Autodesk Fusion 360 part; units mm, degrees
(part 2 of 2)
  point P4 (-72.3362, -41.0103)
  point P5 (-72.5298, -38.3408)
  point P6 (-69.8362, -41.0103)
  point P7 (-69.7968, -38.5103)
  point P8 (-69.7968, -41.0103)
  point P9 (-69.9904, -38.3408)
  point P10 (-67.2968, -41.0103)
  point P11 (-67.2573, -38.5103)
  point P12 (-67.2573, -41.0103)
  point P13 (-67.4509, -38.3408)
  point P14 (-64.7573, -41.0103)
  point P15 (-64.7178, -38.5103)
  point P16 (-64.7178, -41.0103)
  point P17 (-64.9114, -38.3408)
  point P18 (-62.2178, -41.0103)
  point P19 (-62.1783, -38.5103)
  point P20 (-62.1783, -41.0103)
  point P21 (-62.3719, -38.3408)
  point P22 (-59.6783, -41.0103)
  point P23 (-59.6389, -38.5103)
  point P24 (-59.6389, -41.0103)
  point P25 (-59.8325, -38.3408)
  point P26 (-57.1389, -41.0103)
  point P27 (-57.0994, -38.5103)
  point P28 (-57.0994, -41.0103)
  point P29 (-57.293, -38.3408)
  point P30 (-54.5994, -41.0103)
  point P31 (-54.5599, -38.5103)
  point P32 (-54.5599, -41.0103)
  point P33 (-54.7535, -38.3408)
  point P34 (-52.0599, -41.0103)
  point P35 (-52.0204, -38.5103)
  point P36 (-52.0204, -41.0103)
  point P37 (-52.214, -38.3408)
  point P38 (-49.5204, -41.0103)
  point P39 (-49.481, -38.5103)
  point P40 (-49.481, -41.0103)
  point P41 (-49.6746, -38.3408)
  point P42 (-46.981, -41.0103)
  point P43 (-46.9415, -38.5103)
  point P44 (-46.9415, -41.0103)
  point P45 (-47.1351, -38.3408)
  point P46 (-44.4415, -41.0103)
  point P47 (-44.402, -38.5103)
  point P48 (-44.402, -41.0103)
  point P49 (-44.5956, -38.3408)
  point P50 (-41.902, -41.0103)
  point P51 (-41.8626, -38.5103)
  point P52 (-41.8626, -41.0103)
  point P53 (-42.0562, -38.3408)
  point P54 (-39.3626, -41.0103)
  point P55 (-39.3231, -38.5103)
  point P56 (-39.3231, -41.0103)
  point P57 (-39.5167, -38.3408)
  point P58 (-36.8231, -41.0103)
  point P59 (-36.7836, -38.5103)
  point P60 (-36.7836, -41.0103)
  point P61 (-36.9772, -38.3408)
  point P62 (-34.2836, -41.0103)
  point P63 (-34.2441, -38.5103)
  point P64 (-34.2441, -41.0103)
  point P65 (-34.4377, -38.3408)
  point P66 (-31.7441, -41.0103)
  point P67 (-31.7047, -38.5103)
  point P68 (-31.7047, -41.0103)
  point P69 (-31.8983, -38.3408)
  point P70 (-29.2047, -41.0103)
  point P71 (-29.1652, -38.5103)
  point P72 (-29.1652, -41.0103)
  point P73 (-29.3588, -38.3408)
  point P74 (-26.6652, -41.0103)
  point P75 (-26.6257, -38.5103)
  point P76 (-26.6257, -41.0103)
  point P77 (-26.8193, -38.3408)
  point P78 (-24.1257, -41.0103)
  point P79 (-74.8757, -53.8103)
  point P80 (-74.8757, -56.3103)
  point P81 (-75.0693, -53.6408)
  point P82 (-72.3757, -56.3103)
  point P83 (-72.3362, -53.8103)
  point P84 (-72.3362, -56.3103)
  point P85 (-72.5298, -53.6408)
  point P86 (-69.8362, -56.3103)
  point P87 (-69.7968, -53.8103)
  point P88 (-69.7968, -56.3103)
  point P89 (-69.9904, -53.6408)
  point P90 (-67.2968, -56.3103)
  point P91 (-67.2573, -53.8103)
  point P92 (-67.2573, -56.3103)
  point P93 (-67.4509, -53.6408)
  point P94 (-64.7573, -56.3103)
  point P95 (-64.7178, -53.8103)
  point P96 (-64.7178, -56.3103)
  point P97 (-64.9114, -53.6408)
  point P98 (-62.2178, -56.3103)
  point P99 (-62.1783, -53.8103)
  point P100 (-62.1783, -56.3103)
  point P101 (-62.3719, -53.6408)
  point P102 (-59.6783, -56.3103)
  point P103 (-59.6389, -53.8103)
  point P104 (-59.6389, -56.3103)
  point P105 (-59.8325, -53.6408)
  point P106 (-57.1389, -56.3103)
  point P107 (-57.0994, -53.8103)
  point P108 (-57.0994, -56.3103)
  point P109 (-57.293, -53.6408)
  point P110 (-54.5994, -56.3103)
  point P111 (-54.5599, -53.8103)
  point P112 (-54.5599, -56.3103)
  point P113 (-54.7535, -53.6408)
  point P114 (-52.0599, -56.3103)
  point P115 (-52.0204, -53.8103)
  point P116 (-52.0204, -56.3103)
  point P117 (-52.214, -53.6408)
  point P118 (-49.5204, -56.3103)
  point P119 (-49.481, -53.8103)
  point P120 (-49.481, -56.3103)
  point P121 (-49.6746, -53.6408)
  point P122 (-46.981, -56.3103)
  point P123 (-46.9415, -53.8103)
  point P124 (-46.9415, -56.3103)
  point P125 (-47.1351, -53.6408)
  point P126 (-44.4415, -56.3103)
  point P127 (-44.402, -53.8103)
  point P128 (-44.402, -56.3103)
  point P129 (-44.5956, -53.6408)
  point P130 (-41.902, -56.3103)
  point P131 (-41.8626, -53.8103)
  point P132 (-41.8626, -56.3103)
  point P133 (-42.0562, -53.6408)
  point P134 (-39.3626, -56.3103)
  point P135 (-39.3231, -53.8103)
  point P136 (-39.3231, -56.3103)
  point P137 (-39.5167, -53.6408)
  point P138 (-36.8231, -56.3103)
  point P139 (-36.7836, -53.8103)
  point P140 (-36.7836, -56.3103)
  point P141 (-36.9772, -53.6408)
  point P142 (-34.2836, -56.3103)
  point P143 (-34.2441, -53.8103)
  point P144 (-34.2441, -56.3103)
  point P145 (-34.4377, -53.6408)
  point P146 (-31.7441, -56.3103)
  point P147 (-31.7047, -53.8103)
  point P148 (-31.7047, -56.3103)
  point P149 (-31.8983, -53.6408)
  point P150 (-29.2047, -56.3103)
  point P151 (-29.1652, -53.8103)
  point P152 (-29.1652, -56.3103)
  point P153 (-29.3588, -53.6408)
  point P154 (-26.6652, -56.3103)
  point P155 (-26.6257, -53.8103)
  point P156 (-26.6257, -56.3103)
  point P157 (-26.8193, -53.6408)
  point P158 (-24.1257, -56.3103)
  dimension "d61" = 2.5
  dimension "d62" = 2.5
  dimension "d63" = -0.7734
  dimension "d64" = 0.5
  dimension "d67" = 48.25
  dimension "d68" = -15.3
  constraint horizontal L4
  constraint vertical L5
  constraint horizontal L6
  constraint vertical L7
  constraint coincident P2 L6
  constraint coincident P2 L7
  constraint tangent L6 A0
  constraint tangent L7 A0
  constraint tangent L5 A1
  constraint tangent L6 A1
  constraint equal A0 A1
  constraint coincident P1 L4
  constraint coincident P1 L5
  constraint tangent L4 A2
  constraint tangent L5 A2
  constraint equal A0 A2
  constraint coincident P0 L4
  constraint coincident P0 L7
  constraint tangent L4 A3
  constraint tangent L7 A3
  constraint equal A0 A3
  measures "d61" distance of P0 P1
  measures "d62" distance of P0 P2
  measures "d64" radius of A0
extrude "Extrude9" add sketch "Sketch5" along normal blind 2.23 separate body contours L4 L5 L6 L7 A0 A1 A2 A3 | A4 L12 L13 A5 A6 L16 A7 L19 | A8 L20 L21 A9 A10 L24 A11 L27 | A12 L28 L29 A13 A14 L32 A15 L35 | A16 L36 L37 A17 A18 L40 A19 L43 | A20 L44 L45 A21 A22 L48 A23 L51 | A24 L52 L53 A25 A26 L56 A27 L59 | A28 L60 L61 A29 A30 L64 A31 L67 | A32 L68 L69 A33 A34 L72 A35 L75 | A36 L76 L77 A37 A38 L80 A39 L83 | A40 L84 L85 A41 A42 L88 A43 L91 | A44 L92 L93 A45 A46 L96 A47 L99 | A48 L100 L101 A49 A50 L104 A51 L107 | A52 L108 L109 A53 A54 L112 A55 L115 | A56 L116 L117 A57 A58 L120 A59 L123 | A60 L124 L125 A61 A62 L128 A63 L131 | A64 L132 L133 A65 A66 L136 A67 L139 | A68 L140 L141 A69 A70 L144 A71 L147 | A72 L148 L149 A73 A74 L152 A75 L155 | A76 L156 L157 A77 A78 L160 A79 L163 | A80 L164 L165 A81 A82 L168 A83 L171 | A84 L172 L173 A85 A86 L176 A87 L179 | A88 L180 L181 A89 A90 L184 A91 L187 | A92 L188 L189 A93 A94 L192 A95 L195 | A96 L196 L197 A97 A98 L200 A99 L203 | A100 L204 L205 A101 A102 L208 A103 L211 | A104 L212 L213 A105 A106 L216 A107 L219 | A108 L220 L221 A109 A110 L224 A111 L227 | A112 L228 L229 A113 A114 L232 A115 L235 | A116 L236 L237 A117 A118 L240 A119 L243 | A120 L244 L245 A121 A122 L248 A123 L251 | A124 L252 L253 A125 A126 L256 A127 L259 | A128 L260 L261 A129 A130 L264 A131 L267 | A132 L268 L269 A133 A134 L272 A135 L275 | A136 L276 L277 A137 A138 L280 A139 L283 | A140 L284 L285 A141 A142 L288 A143 L291 | A144 L292 L293 A145 A146 L296 A147 L299 | A148 L300 L301 A149 A150 L304 A151 L307 | A152 L308 L309 A153 A154 L312 A155 L315 | A156 L316 L317 A157 A158 L320 A159 L323 makes body 21 at (-69.539, 39.6015, 0) makes body 22 at (-59.3811, 39.6015, 0) makes body 23 at (-48.0721, 38.7682, 0) makes body 24 at (-39.0653, 39.6015, 0) makes body 25 at (-28.074, 38.7682, 0) makes body 26 at (-31.4469, 54.9015, 0) makes body 27 at (-41.6047, 54.9015, 0) makes body 28 at (-49.7783, 54.9015, 0) makes body 29 at (-61.9205, 54.9015, 0) makes body 30 at (-72.0784, 54.9015, 0) makes body 31 at (-69.539, 54.9015, 0) makes body 32 at (-59.3811, 54.9015, 0) makes body 33 at (-47.2388, 54.9015, 0) makes body 34 at (-39.0653, 54.9015, 0) makes body 35 at (-28.9074, 54.9015, 0) makes body 36 at (-30.6135, 38.7682, 0) makes body 37 at (-40.7714, 38.7682, 0) makes body 38 at (-49.7783, 39.6015, 0) makes body 39 at (-61.9205, 39.6015, 0) makes body 40 at (-72.0784, 39.6015, 0) makes body 41 at (-66.9995, 39.6015, 0) makes body 42 at (-56.0083, 38.7682, 0) makes body 43 at (-44.6993, 39.6015, 0) makes body 44 at (-36.5258, 39.6015, 0) makes body 45 at (-25.5346, 38.7682, 0) makes body 46 at (-33.9863, 54.9015, 0) makes body 47 at (-44.1442, 54.9015, 0) makes body 48 at (-54.3021, 54.9015, 0) makes body 49 at (-64.46, 54.9015, 0) makes body 50 at (-74.6179, 54.9015, 0) makes body 51 at (-66.9995, 54.9015, 0) makes body 52 at (-56.8416, 54.9015, 0) makes body 53 at (-44.6993, 54.9015, 0) makes body 54 at (-36.5258, 54.9015, 0) makes body 55 at (-26.3679, 54.9015, 0) makes body 56 at (-33.9863, 39.6015, 0) makes body 57 at (-44.1442, 39.6015, 0) makes body 58 at (-54.3021, 39.6015, 0) makes body 59 at (-64.46, 39.6015, 0) makes body 60 at (-74.6179, 39.6015, 0)
extrude "Extrude10" add sketch "Sketch5" along normal blind 8.5 separate body contours L8 L9 L10 L11 | L14 L15 L17 L18 | L22 L23 L25 L26 | L30 L31 L33 L34 | L38 L39 L41 L42 | L46 L47 L49 L50 | L54 L55 L57 L58 | L62 L63 L65 L66 | L70 L71 L73 L74 | L78 L79 L81 L82 | L86 L87 L89 L90 | L94 L95 L97 L98 | L102 L103 L105 L106 | L110 L111 L113 L114 | L118 L119 L121 L122 | L126 L127 L129 L130 | L134 L135 L137 L138 | L142 L143 L145 L146 | L150 L151 L153 L154 | L158 L159 L161 L162 | L166 L167 L169 L170 | L174 L175 L177 L178 | L182 L183 L185 L186 | L190 L191 L193 L194 | L198 L199 L201 L202 | L206 L207 L209 L210 | L214 L215 L217 L218 | L222 L223 L225 L226 | L230 L231 L233 L234 | L238 L239 L241 L242 | L246 L247 L249 L250 | L254 L255 L257 L258 | L262 L263 L265 L266 | L270 L271 L273 L274 | L278 L279 L281 L282 | L286 L287 L289 L290 | L294 L295 L297 L298 | L302 L303 L305 L306 | L310 L311 L313 L314 | L318 L319 L321 L322 makes body 61 at (-29.9781, 39.9192, -2.8333) makes body 62 at (-40.136, 39.9192, -2.8333) makes body 63 at (-50.2939, 39.9192, -2.8333) makes body 64 at (-60.4518, 39.9192, -2.8333) makes body 65 at (-70.6097, 39.9192, -2.8333) makes body 66 at (-68.0702, 55.2192, -2.8333) makes body 67 at (-57.9123, 55.2192, -2.8333) makes body 68 at (-47.7544, 55.2192, -2.8333) makes body 69 at (-37.5965, 55.2192, -2.8333) makes body 70 at (-27.4386, 55.2192, -2.8333) makes body 71 at (-29.9781, 55.2192, -2.8333) makes body 72 at (-40.136, 55.2192, -2.8333) makes body 73 at (-50.2939, 55.2192, -2.8333) makes body 74 at (-60.4518, 55.2192, -2.8333) makes body 75 at (-70.6097, 55.2192, -2.8333) makes body 76 at (-68.0702, 39.9192, -2.8333) makes body 77 at (-57.9123, 39.9192, -2.8333) makes body 78 at (-47.7544, 39.9192, -2.8333) makes body 79 at (-37.5965, 39.9192, -2.8333) makes body 80 at (-27.4386, 39.9192, -2.8333) makes body 81 at (-32.5176, 39.9192, -2.8333) makes body 82 at (-42.6755, 39.9192, -2.8333) makes body 83 at (-52.8333, 39.9192, -2.8333) makes body 84 at (-62.9912, 39.9192, -2.8333) makes body 85 at (-74.1023, 39.6015, -2.8333) makes body 86 at (-65.5307, 55.2192, -2.8333) makes body 87 at (-55.3728, 55.2192, -2.8333) makes body 88 at (-45.2149, 55.2192, -2.8333) makes body 89 at (-35.057, 55.2192, -2.8333) makes body 90 at (-24.8991, 55.2192, -2.8333) makes body 91 at (-32.5176, 55.2192, -2.8333) makes body 92 at (-42.6755, 55.2192, -2.8333) makes body 93 at (-52.8333, 55.2192, -2.8333) makes body 94 at (-62.9912, 55.2192, -2.8333) makes body 95 at (-73.1491, 55.2192, -2.8333) makes body 96 at (-65.5307, 39.9192, -2.8333) makes body 97 at (-55.3728, 39.9192, -2.8333) makes body 98 at (-45.2149, 39.9192, -2.8333) makes body 99 at (-35.057, 39.9192, -2.8333) makes body 100 at (-24.8991, 39.9192, -2.8333)
chamfer "Chamfer1" distance 0.3 angle 45 40 faces at (-71.2451, 39.6015, -8.5) (-50.9293, 39.6015, -8.5) (-30.6135, 39.6015, -8.5) (-61.0872, 39.6015, -8.5) (-40.7714, 39.6015, -8.5) (-68.7056, 54.9015, -8.5) (-68.7056, 39.6015, -8.5) (-50.9293, 54.9015, -8.5) (-61.0872, 54.9015, -8.5) (-58.5477, 39.6015, -8.5) (-71.2451, 54.9015, -8.5) (-48.3898, 39.6015, -8.5) (-30.6135, 54.9015, -8.5) (-40.7714, 54.9015, -8.5) (-38.2319, 54.9015, -8.5) (-58.5477, 54.9015, -8.5) (-48.3898, 54.9015, -8.5) (-28.074, 54.9015, -8.5) (-53.4688, 39.6015, -8.5) (-63.6267, 39.6015, -8.5) (-38.2319, 39.6015, -8.5) (-28.074, 39.6015, -8.5) (-43.3109, 39.6015, -8.5) (-33.153, 39.6015, -8.5) (-56.0083, 54.9015, -8.5) (-45.8504, 54.9015, -8.5) (-73.7846, 39.6015, -8.5) (-35.6925, 54.9015, -8.5) (-25.5346, 54.9015, -8.5) (-66.1661, 54.9015, -8.5) (-63.6267, 54.9015, -8.5) (-73.7846, 54.9015, -8.5) (-66.1661, 39.6015, -8.5) (-43.3109, 54.9015, -8.5) (-33.153, 54.9015, -8.5) (-53.4688, 54.9015, -8.5) (-45.8504, 39.6015, -8.5) (-56.0083, 39.6015, -8.5) (-35.6925, 39.6015, -8.5) (-25.5346, 39.6015, -8.5) on bodies 61 62 63 64 65 66 67 68 69 70 71 72 73 74 75 76 77 78 79 80 81 82 83 84 85 86 87 88 89 90 91 92 93 94 95 96 97 98 99 100
chamfer "Chamfer2" distance 0.2 angle 45 10 faces at (-62.1731, 46.7774, 7.53) (-60.9231, 48.2774, 7.53) (-64.8398, 48.2774, 7.53) (-63.4231, 46.7774, 7.53) (-62.1731, 48.2774, 7.53) (-64.8398, 46.7774, 7.53) (-63.4231, 48.2774, 7.53) (-60.9231, 46.7774, 7.53) (-66.0898, 46.7774, 7.53) (-65.9231, 48.1107, 7.53) on bodies 7 8 9 10 11 12 13 14 15 16
extrude "Extrude11" add sketch "Sketch5" against normal blind 3 separate body contours L8 L9 L10 L11 | L14 L15 L17 L18 | L22 L23 L25 L26 | L30 L31 L33 L34 | L38 L39 L41 L42 | L46 L47 L49 L50 | L54 L55 L57 L58 | L62 L63 L65 L66 | L70 L71 L73 L74 | L78 L79 L81 L82 | L86 L87 L89 L90 | L94 L95 L97 L98 | L102 L103 L105 L106 | L110 L111 L113 L114 | L118 L119 L121 L122 | L126 L127 L129 L130 | L134 L135 L137 L138 | L142 L143 L145 L146 | L150 L151 L153 L154 | L158 L159 L161 L162 | L166 L167 L169 L170 | L174 L175 L177 L178 | L182 L183 L185 L186 | L190 L191 L193 L194 | L198 L199 L201 L202 | L206 L207 L209 L210 | L214 L215 L217 L218 | L222 L223 L225 L226 | L230 L231 L233 L234 | L238 L239 L241 L242 | L246 L247 L249 L250 | L254 L255 L257 L258 | L262 L263 L265 L266 | L270 L271 L273 L274 | L278 L279 L281 L282 | L286 L287 L289 L290 | L294 L295 L297 L298 | L302 L303 L305 L306 | L310 L311 L313 L314 | L318 L319 L321 L322 makes body 101 at (-29.9781, 39.9192, 1) makes body 102 at (-40.136, 39.9192, 1) makes body 103 at (-50.2939, 39.9192, 1) makes body 104 at (-60.4518, 39.9192, 1) makes body 105 at (-70.6097, 39.9192, 1) makes body 106 at (-29.9781, 55.2192, 1) makes body 107 at (-40.136, 55.2192, 1) makes body 108 at (-50.2939, 55.2192, 1) makes body 109 at (-60.4518, 55.2192, 1) makes body 110 at (-70.6097, 55.2192, 1) makes body 111 at (-68.0702, 55.2192, 1) makes body 112 at (-57.9123, 55.2192, 1) makes body 113 at (-47.7544, 55.2192, 1) makes body 114 at (-37.5965, 55.2192, 1) makes body 115 at (-27.4386, 55.2192, 1) makes body 116 at (-68.0702, 39.9192, 1) makes body 117 at (-57.9123, 39.9192, 1) makes body 118 at (-47.7544, 39.9192, 1) makes body 119 at (-37.5965, 39.9192, 1) makes body 120 at (-27.4386, 39.9192, 1) makes body 121 at (-32.5176, 39.9192, 1) makes body 122 at (-42.6755, 39.9192, 1) makes body 123 at (-52.8333, 39.9192, 1) makes body 124 at (-62.9912, 39.9192, 1) makes body 125 at (-74.1023, 39.6015, 1) makes body 126 at (-32.5176, 55.2192, 1) makes body 127 at (-42.6755, 55.2192, 1) makes body 128 at (-52.8333, 55.2192, 1) makes body 129 at (-62.9912, 55.2192, 1) makes body 130 at (-73.1491, 55.2192, 1) makes body 131 at (-65.5307, 55.2192, 1) makes body 132 at (-55.3728, 55.2192, 1) makes body 133 at (-45.2149, 55.2192, 1) makes body 134 at (-35.057, 55.2192, 1) makes body 135 at (-24.8991, 55.2192, 1) makes body 136 at (-65.5307, 39.9192, 1) makes body 137 at (-55.3728, 39.9192, 1) makes body 138 at (-45.2149, 39.9192, 1) makes body 139 at (-35.057, 39.9192, 1) makes body 140 at (-24.8991, 39.9192, 1)
fillet "Fillet3" radius 0.35 40 faces at (-30.6135, 39.6015, 3) (-40.7714, 39.6015, 3) (-50.9293, 39.6015, 3) (-61.0872, 39.6015, 3) (-71.2451, 39.6015, 3) (-30.6135, 54.9015, 3) (-40.7714, 54.9015, 3) (-50.9293, 54.9015, 3) (-61.0872, 54.9015, 3) (-71.2451, 54.9015, 3) (-68.7056, 54.9015, 3) (-58.5477, 54.9015, 3) (-48.3898, 54.9015, 3) (-38.2319, 54.9015, 3) (-28.074, 54.9015, 3) (-68.7056, 39.6015, 3) (-58.5477, 39.6015, 3) (-48.3898, 39.6015, 3) (-38.2319, 39.6015, 3) (-28.074, 39.6015, 3) (-33.153, 39.6015, 3) (-43.3109, 39.6015, 3) (-53.4688, 39.6015, 3) (-63.6267, 39.6015, 3) (-73.7846, 39.6015, 3) (-33.153, 54.9015, 3) (-43.3109, 54.9015, 3) (-53.4688, 54.9015, 3) (-63.6267, 54.9015, 3) (-73.7846, 54.9015, 3) (-66.1661, 54.9015, 3) (-56.0083, 54.9015, 3) (-45.8504, 54.9015, 3) (-35.6925, 54.9015, 3) (-25.5346, 54.9015, 3) (-66.1661, 39.6015, 3) (-56.0083, 39.6015, 3) (-45.8504, 39.6015, 3) (-35.6925, 39.6015, 3) (-25.5346, 39.6015, 3) on bodies 101 102 103 104 105 106 107 108 109 110 111 112 113 114 115 116 117 118 119 120 121 122 123 124 125 126 127 128 129 130 131 132 133 134 135 136 137 138 139 140
sketch "Sketch6" plane through (-76.5893, 0, 0) normal (-1, 0, 0) x (0, -1, 0)
  arc A0 (-43.9208, 4.03) -> (-44.1208, 4.23) centre (-44.1208, 4.03) ccw
  line L0 (-43.9208, 4.03) -> (-43.9208, 1.83)
  line L1 (-43.9208, 1.83) -> (-50.8708, 1.83)
  line L2 (-50.8708, 1.83) -> (-50.8708, 4.03)
  arc A1 (-50.6708, 4.23) -> (-50.8708, 4.03) centre (-50.6708, 4.03) ccw
  line L3 (-50.6708, 4.23) -> (-44.1208, 4.23)
  arc A2 (-43.6208, 4.03) -> (-44.1208, 4.53) centre (-44.1208, 4.03) ccw
  line L4 (-44.1208, 4.53) -> (-50.6708, 4.53)
  arc A3 (-50.6708, 4.53) -> (-51.1708, 4.03) centre (-50.6708, 4.03) ccw
  line L5 (-51.1708, 4.03) -> (-51.1708, 1.53)
  line L6 (-51.1708, 1.53) -> (-43.6208, 1.53)
  line L7 (-43.6208, 1.53) -> (-43.6208, 4.03)
  arc A4 (-50.6708, 4.53) -> (-51.1708, 4.03) centre (-50.6708, 4.03) ccw
  line L8 (-51.1708, 1.53) -> (-51.1708, 4.03)
  line L9 (-43.6208, 1.53) -> (-43.6208, 4.03)
  arc A5 (-43.6208, 4.03) -> (-44.1208, 4.53) centre (-44.1208, 4.03) ccw
  line L10 (-50.6708, 4.53) -> (-44.1208, 4.53)
  line L11 (-51.4208, 4.03) -> (-51.4208, 1.28)
  line L12 (-51.4208, 1.28) -> (-43.3708, 1.28)
  line L13 (-43.3708, 1.28) -> (-43.3708, 4.03)
  arc A6 (-43.3708, 4.03) -> (-44.1208, 4.78) centre (-44.1208, 4.03) ccw
  line L14 (-44.1208, 4.78) -> (-50.6708, 4.78)
  arc A7 (-50.6708, 4.78) -> (-51.4208, 4.03) centre (-50.6708, 4.03) ccw
  dimension "d79" = 0.25
extrude "Extrude12" add sketch "Sketch6" against normal blind 0.25 contours L11 L12 L13 A6 L14 A7 bodies 6
fillet "Fillet4" radius 0.15 5 edges at (-76.3393, 51.1708, 2.78) (-76.3393, 51.0243, 4.3836) (-76.3393, 47.3958, 4.53) (-76.3393, 43.7672, 4.3836) (-76.3393, 43.6208, 2.78) on bodies 6
fillet "Fillet5" radius 0.3 6 edges at (-76.5893, 50.8708, 2.93) (-76.5893, 50.8122, 4.1714) (-76.5893, 47.3958, 4.23) (-76.5893, 43.9793, 4.1714) (-76.5893, 43.9208, 2.93) (-76.5893, 47.3958, 1.83) on bodies 6
equation "d17 = ( 4.3 / 2 ) * 1 mm"
equation "d18 = ( 4.3 / 2 ) * 1 mm"
equation "d19 = ( 13 / 2 ) * 1 mm"
equation "d20 = ( 13 / 2 ) * 1 mm"
equation "d21 = ( 10.04 / 2 ) * 1 mm"
equation "d22 = ( 10.04 / 2 ) * 1 mm"
equation "d23 = ( 3.36 / 2 ) * 1 mm"
equation "d24 = ( 3.36 / 2 ) * 1 mm"
equation "d25 = ( 7.55 / 2 ) * 1 mm"
equation "d26 = ( 7.55 / 2 ) * 1 mm"
